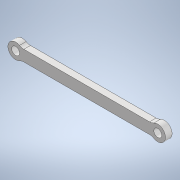
# Autodesk Inventor part: ff2
Saved by Autodesk Inventor 2020 (Build 240168000, 168)
## iProperties
Created: 2020-11-09
Part Number: ff2
Material: Generic
Document SubType Name: Modeling
Designer: alnwlsn
Density: 1 g/cm^3
Appearance: Default
Author: alnwlsn
Autodesk Inventor part; units mm, degrees
ref_plane "YZ Plane" through (0, 0, 0) normal (1, 0, 0) x (0, 1, 0)
ref_plane "XZ Plane" through (0, 0, 0) normal (0, 1, 0) x (-1, 0, 0)
ref_plane "XY Plane" through (0, 0, 0) normal (0, 0, 1) x (1, 0, 0)
sketch "Sketch1" plane through (0, 0, 0) normal (0, 0, 1) x (1, 0, 0)
  circle A0 centre (0, 0) radius 1
  circle A1 centre (0, 0) radius 2
  line L0 (0, 0) -> (32.3, 0) construction
  circle A2 centre (32.3, 0) radius 2
  circle A3 centre (32.3, 0) radius 1
  line L1 (1, 1.5) -> (31.3, 1.5)
  line L2 (31.3, 1.5) -> (31.3, -1.5)
  line L3 (31.3, -1.5) -> (1, -1.5)
  line L4 (1, -1.5) -> (1, 1.5)
  line L5 (1, 1.5) -> (31.3, -1.5) construction
  line L6 (31.3, 1.5) -> (1, -1.5) construction
  point P0 (16.15, 0)
  point P1 (1.3229, -1.5)
  point P2 (30.9771, -1.5)
  point P3 (30.9771, 1.5)
  point P4 (1.3229, 1.5)
  dimension "d0" = 2
  dimension "d1" = 4
  dimension "d8" = 3
  dimension "d9" = 32.3
  constraints: 14 end point, 4 centre point, 4 coincident, 3 midpoint, 2 equal radius, 2 horizontal, 2 parallel, 1 perpendicular, 1 tangent
  measures "d0" diameter of A0
  measures "d1" diameter of A1
  measures "d8" distance between parallel lines of L3 L1
  measures "d9" distance of point (0, 0) L0.end
extrude "Extrusion1" add sketch "Sketch1" along normal blind 1.5
fillet "Fillet2" radius 2 4 edges at (1.3229, 1.5, 0.75) (30.9771, 1.5, 0.75) (30.9771, -1.5, 0.75) (1.3229, -1.5, 0.75)
body "Solid1"
